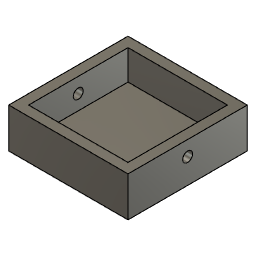
base v2 (Autodesk Fusion 360 design; units mm, degrees)
Autodesk Fusion 360 part; units mm, degrees
sketch "Sketch1" plane through (0, 0, 0) normal (1, 0, 0) x (0, 0, -1)
sketch "Sketch2" plane through (0, 0, 0) normal (0, 1, 0) x (1, 0, 0)
  line L0 (0, 0) -> (50, 0)
  line L1 (50, 0) -> (50, 50)
  line L2 (50, 50) -> (0, 50)
  line L3 (0, 50) -> (0, 0)
  line L4 (-5, -5) -> (55, -5)
  line L5 (55, -5) -> (55, 55)
  line L6 (55, 55) -> (-5, 55)
  line L7 (-5, 55) -> (-5, -5)
  dimension "d1" = 50
  dimension "d2" = 50
  dimension "d3" = 5
  constraint horizontal L0
  constraint vertical L1
  constraint horizontal L2
  constraint vertical L3
  constraint coincident L0.start L3.end
  measures "d1" distance of L0.start L0.end
  measures "d2" distance of L0.start L2.end
extrude "Extrude1" add sketch "Sketch2" along normal blind 20
extrude "Extrude2" add sketch "Sketch2" along normal blind 5 contours L0 L1 L2 L3
sketch "Sketch3" plane through (-5, 0, 0) normal (-1, 0, 0) x (0, 0, 1)
  line L0 (-55, 0) -> (5, 0)
  line L1 (5, 0) -> (5, 20)
  line L2 (5, 20) -> (-55, 20)
  line L3 (-55, 20) -> (-55, 0)
  line L4 (-25, 20) -> (-25, 12.5) construction
  circle A0 centre (-25, 12.5) radius 2.5
  dimension "d8" = 7.5
  dimension "d9" = 5
  constraint midpoint L2 L4.start
  constraint perpendicular L2 L4
  constraint coincident L4.end A0.centre
  measures "d8" distance of L4.start L4.end
  measures "d9" diameter of A0
extrude "Extrude3" cut sketch "Sketch3" against normal blind 163 contours A0
